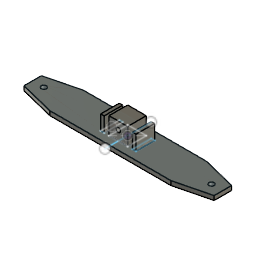
Support_boite_capteur_bras (Autodesk Fusion 360 design; units mm, degrees)
Autodesk Fusion 360 part; units mm, degrees
note: some values were not read from the file. Chosen so that the rebuilt part matches the saved one: a direction; which face or edge a step refers to. Set by a fixed rule: which sketch regions a step uses.
sketch "Esquisse1" plane through (0, 0, 0) normal (0, 0, 1) x (1, 0, 0)
  line L0 (-35.5672, 10) -> (35.5672, 10)
  line L1 (55, 5.1418) -> (55, -5)
  line L2 (35, -10) -> (-35, -10)
  line L3 (-55, -5) -> (-55, 5.1418)
  line L4 (-55, 10) -> (55, -10) construction
  line L5 (55, 10) -> (-55, -10) construction
  circle A0 centre (48.5, 0) radius 1.5
  circle A1 centre (-48.5, 0) radius 1.5
  line L6 (-35, -10) -> (-55, -5)
  line L7 (-60.655, 0.0709) -> (59.7352, 0.0709)
  line L8 (-35, 10.1418) -> (-55, 5.1418)
  line L9 (0, -15.9184) -> (0, 14.9181)
  line L10 (35, 10.1418) -> (55, 5.1418)
  line L11 (35, -10) -> (55, -5)
  dimension "d1" = 110
  dimension "d2" = 20
  dimension "d3" = 3
  dimension "d4" = 3
  dimension "d5" = 97
  dimension "d6" = 6.5
  dimension "d9" = 20
  dimension "d10" = 5
  constraint horizontal L0
  constraint perpendicular L0 L1
  constraint parallel L0 L2
  constraint parallel L1 L3
  constraint coincident L4 origin
  constraint coincident L5 origin
  constraint horizontal L7
  constraint symmetric L2.end L7 L8.start
  constraint symmetric L3.start L7 L3.end
  constraint perpendicular L0 L9
  constraint symmetric L2.end L9 L2.start
  constraint symmetric L3.start L9 L1.end
  constraint symmetric L8.start L9 L10.start
  constraint symmetric L3.end L9 L1.start
  constraint coincident L8 L0.start
  constraint coincident L10 L0.end
  measures "d1" distance of L4.end L5.end
  measures "d2" distance of L5.start L4.end
  measures "d3" diameter of A0
  measures "d4" diameter of A1
  measures "d5" distance of A0.centre A1.centre
  measures "d6" distance of L1 A0.centre
  measures "d9" distance of L5.end L2.end
  measures "d10" distance of L5.end L3.start
extrude "Extrusion1" add sketch "Esquisse1" along normal blind 2.5 contours L0 L3 A1 L7 L8 L9 | L0 L1 A0 L7 L9 L10 | L2 L3 A1 L6 L7 L9 | L1 L2 A0 L7 L9 L11
sketch "Esquisse2" plane through (0, 0, 2.5) normal (0, 0, 1) x (-1, 0, 0)
  circle A0 centre (-48.5, 0) radius 1.5
  circle A1 centre (48.5, 0) radius 1.5
  line L0 (35, 10) -> (-35, 10)
  line L1 (-35, 10) -> (-55, 5)
  line L2 (-55, 5) -> (-55, -5.1418)
  line L3 (-55, -5.1418) -> (-35.5672, -10)
  line L4 (-35.5672, -10) -> (35.5672, -10)
  line L5 (35.5672, -10) -> (55, -5.1418)
  line L6 (55, -5.1418) -> (55, 5)
  line L7 (55, 5) -> (35, 10)
  line L8 (5.4, -5.4) -> (-5.4, -5.4)
  line L9 (-5.4, -5.4) -> (-5.4, 5.4)
  line L10 (-5.4, 5.4) -> (5.4, 5.4)
  line L11 (5.4, 5.4) -> (5.4, -5.4)
  line L12 (5.4, -5.4) -> (-5.4, 5.4) construction
  line L13 (-5.4, -5.4) -> (5.4, 5.4) construction
  line L14 (10.2, -5.4) -> (8.2, -5.4)
  line L15 (8.2, -5.4) -> (8.2, 5.4)
  line L16 (8.2, 5.4) -> (10.2, 5.4)
  line L17 (10.2, 5.4) -> (10.2, -5.4)
  line L18 (10.2, -5.4) -> (8.2, 5.4) construction
  line L19 (8.2, -5.4) -> (10.2, 5.4) construction
  line L20 (0, -13.4838) -> (0, 13.0906)
  line L21 (-8.2, -5.4) -> (-10.2, 5.4) construction
  line L22 (-10.2, -5.4) -> (-8.2, 5.4) construction
  line L23 (-10.2, -5.4) -> (-8.2, -5.4)
  line L24 (-8.2, -5.4) -> (-8.2, 5.4)
  line L25 (-8.2, 5.4) -> (-10.2, 5.4)
  line L26 (-10.2, 5.4) -> (-10.2, -5.4)
  point P0 (9.2, 0)
  dimension "d11" = 10.8
  dimension "d12" = 10.8
  dimension "d13" = 2
  dimension "d14" = 10.8
  dimension "d15" = 2.8
  constraint horizontal L8
  constraint perpendicular L8 L9
  constraint parallel L8 L10
  constraint parallel L9 L11
  constraint coincident L12 origin
  constraint coincident L13 origin
  constraint horizontal L14
  constraint perpendicular L14 L15
  constraint parallel L14 L16
  constraint parallel L15 L17
  constraint coincident L18 P0
  constraint coincident L19 P0
  constraint perpendicular L0 L20
  constraint symmetric L14.start L20 L22.start
  constraint symmetric L14.end L20 L21.start
  constraint symmetric L15.end L20 L22.end
  constraint symmetric L16.end L20 L21.end
  measures "d11" distance of L9.end L10.end
  measures "d12" distance of L8.end L9.end
  measures "d13" distance of L15.end L16.end
  measures "d14" distance of L14.end L15.end
  measures "d15" distance of L11 L15
extrude "Extrusion2" add sketch "Esquisse2" along normal blind 10 contours L8 L9 L10 L20 | L8 L10 L11 L20
sketch "Esquisse3" plane through (0, 5.4, 0) normal (0, 1, 0) x (-1, 0, 0)
  line L0 (-5.4, 2.5) -> (5.4, 2.5)
  line L1 (5.4, 2.5) -> (5.4, 12.5)
  line L2 (5.4, 12.5) -> (-5.4, 12.5)
  line L3 (-5.4, 12.5) -> (-5.4, 2.5)
  circle A0 centre (0, 8) radius 1.25
  line L4 (-35.5672, 2.5) -> (35.5672, 2.5)
  dimension "d18" = 2.5
  dimension "d19" = 5.5
  measures "d18" diameter of A0
  measures "d19" distance of A0.centre L4
extrude "Extrusion3" cut sketch "Esquisse3" against normal through all contours A0
extrude "Extrusion4" add sketch "Esquisse2" along normal blind 8.5 contours L14 L15 L16 L17 | L23 L24 L25 L26
